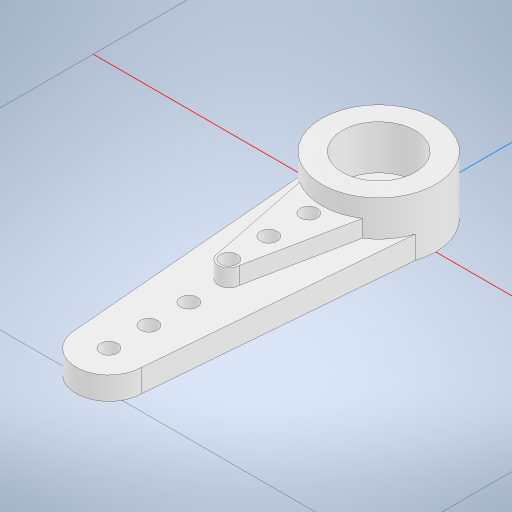
# Autodesk Inventor part: weißes_ding
Saved by Autodesk Inventor 2023 (Build 270158000, 158)
## iProperties
Created: 2022-06-22
Part Number: weißes_ding
Material: Plastic, Opaque White
Document SubType Name: Modeling
Designer: dennis
Density: 0.952 g/cm^3
Appearance: Smooth - White
Mass: 0.315326 g
Surface Area: 5.51546 cm^2
Volume: 0.315326 cm^3
Author: dennis
Autodesk Inventor part; units mm, degrees
ref_plane "YZ Plane" through (0, 0, 0) normal (1, 0, 0) x (0, 1, 0)
ref_plane "XZ Plane" through (0, 0, 0) normal (0, 1, 0) x (-1, 0, 0)
ref_plane "XY Plane" through (0, 0, 0) normal (0, 0, 1) x (1, 0, 0)
sketch "Skizze1" plane through (0, 0, 0) normal (0, 1, 0) x (-1, 0, 0)
  circle A0 centre (0, 0) radius 4
  circle A1 centre (0, 0) radius 1.25
  line L0 (0, -4) -> (0, 21.2)
  line L1 (0, 21.2) -> (0, 18.9)
  circle A2 centre (0, 18.9) radius 0.6
  circle A3 centre (0, 18.9) radius 2.3
  line L2 (0, 18.9) -> (0, 16.1)
  line L3 (0, 16.1) -> (0, 13.3)
  circle A4 centre (0, 16.1) radius 0.6
  line L4 (0, 16.1) -> (0, 13.3)
  circle A5 centre (0, 13.3) radius 0.6
  line L5 (0, 13.3) -> (0, 10.5)
  circle A6 centre (0, 10.5) radius 0.6
  line L6 (0, 10.5) -> (0, 7.7)
  circle A7 centre (0, 7.7) radius 0.6
  line L7 (0, 7.7) -> (0, 4.9)
  circle A8 centre (0, 4.9) radius 0.6
  circle A9 centre (0, 10.5) radius 0.75
  line L8 (0.75, 10.5) -> (2.2, 3.3407)
  line L9 (-0.75, 10.5) -> (-2.2, 3.3407)
  circle A10 centre (0, 0) radius 2.95
  circle A11 centre (0, 0) radius 2.55
  line L10 (-3.7997, 1.25) -> (-2.3, 18.9)
  line L11 (3.7997, 1.25) -> (2.3, 18.9)
  point P0 (-4, 0)
  point P1 (4, 0)
  point P2 (0.3, 16.6196)
  point P3 (-0.3, 16.6196)
  dimension "d0" = 8
  dimension "d2" = 2.5
  dimension "d4" = 25.2
  dimension "d5" = 2.3
  dimension "d6" = 1.2
  dimension "d7" = 2.8
  dimension "d10" = 1.2
  dimension "d11" = 2.8
  dimension "d12" = 1.2
  dimension "d13" = 2.8
  dimension "d14" = 1.2
  dimension "d15" = 2.8
  dimension "d16" = 1.2
  dimension "d17" = 2.8
  dimension "d18" = 1.2
  dimension "d19" = 1.5
  dimension "d20" = 5.9
  dimension "d21" = 5.1
  constraints: 24 end point, 12 coincident, 11 centre point, 6 point on circle, 6 point on line, 1 collinear, 1 vertical, 9 other
  measures "d2" diameter of A1
  measures "d4" distance of L0.start L0.end
  measures "d5" distance of L0.end L1.end
  measures "d6" diameter of A2
  measures "d7" distance of L2.start L2.end
  measures "d10" diameter of A4
  measures "d11" distance of L4.start L3.end
  measures "d12" diameter of A5
  measures "d13" distance of L5.start L5.end
  measures "d14" diameter of A6
  measures "d15" distance of L6.start L6.end
  measures "d16" diameter of A7
  measures "d17" distance of L7.start L7.end
  measures "d18" diameter of A8
  measures "d19" diameter of A9
  measures "d20" diameter of A10
  measures "d21" diameter of A11
extrude "Extrusion1" add sketch "Skizze1" along normal blind 1.6 contours A0 L0 A10 | A0 L8 A9 L0 A5 A4 A3 L11 | A0 L0 A10 | A0 L0 A8 A7 A9 L8 | A3 A4 L0 A2 | L10 A3 A4 L0 A5 A9 L9 A0 | A10 L0 A11 | L0 A11 A10 | A0 L9 A9 L0 A7 A8 | A9 L0 A6 | L0 A2 A4 A3 | L0 A6 A9
extrude "Extrusion2" add sketch "Skizze1" along normal blind 2.8 contours A0 L0 A10 | A0 L0 A10 | A0 L0 A8 A7 A9 L8 | A10 L0 A11 | L0 A11 A10 | A0 L9 A9 L0 A7 A8 | A9 L0 A6 | L0 A6 A9
extrude "Extrusion3" add sketch "Skizze1" along normal blind 4.1 contours A0 L0 A10 | A0 L0 A10 | A10 L0 A11 | L0 A11 A10
extrude "Extrusion4" add sketch "Skizze1" along normal blind 1 contours A11 L0 A1 | L0 A1 A11
extrude "Extrusion5" cut sketch "Skizze1" along normal blind 0.5 contours A10 L0 A11 | L0 A11 A10 | A11 L0 A1 | L0 A1 A11
